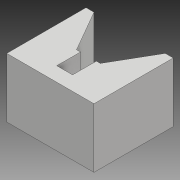
# Autodesk Inventor part: soporte_antena_aquiles
Saved by Autodesk Inventor 2018 (Build 220112000, 112)
## iProperties
Created: 2019-01-15
Part Number: soporte_antena_aquiles
Material: Genérico
Document SubType Name: Modeling
Designer: becar
Density: 1 g/cm^3
Appearance: Valor por defecto
Author: becar
Autodesk Inventor part; units mm, degrees
ref_plane "YZ Plane" through (0, 0, 0) normal (1, 0, 0) x (0, 1, 0)
ref_plane "XZ Plane" through (0, 0, 0) normal (0, 1, 0) x (-1, 0, 0)
ref_plane "XY Plane" through (0, 0, 0) normal (0, 0, 1) x (1, 0, 0)
sketch "Boceto1" plane through (0, 0, 0) normal (0, 0, 1) x (1, 0, 0)
  line L0 (0, 0) -> (0, 15)
  line L1 (0, 15) -> (2, 15)
  line L2 (2, 15) -> (8, 4.6077)
  line L3 (2, 15) -> (14, 15) construction
  line L4 (0, 0) -> (0, -5)
  line L5 (8, 4.6077) -> (14, 4.6077)
  line L6 (14, 4.6077) -> (20, 15)
  line L7 (20, 15) -> (22, 15)
  line L8 (22, 15) -> (22, -0.0111)
  line L9 (22, -0.0111) -> (22, -5)
  line L10 (22, -5) -> (0, -5)
  dimension "d0" = 15
  dimension "d1" = 2
  dimension "d2" = 12
  dimension "d3" = 60
  dimension "d4" = 5
  dimension "d5" = 6
  dimension "d6" = 12
  dimension "d7" = 2
  constraints: 22 end point, 3 perpendicular, 2 horizontal, 2 vertical, 1 equal length, 1 parallel, 1 point on line
  measures "d0" distance of L0.start L0.end
  measures "d1" distance of L0.end L1.end
  measures "d2" distance of L1.end L2.end
  measures "d3" angle of L2 L3
  measures "d4" distance of L0.start L4.end
  measures "d5" distance of L2.end L5.end
  measures "d6" distance of L5.end L6.end
  measures "d7" distance of L6.end L7.end
extrude "Extrusión1" add sketch "Boceto1" along normal blind 15
sketch "Boceto2" plane through (0, 0, 15) normal (0, 0, 1) x (1, 0, 0)
  line L0 (14, 4.6077) -> (8, 4.6077) projected
  line L1 (8, 4.6077) -> (9, 4.6077)
  line L2 (9, 4.6077) -> (9, -1.3923)
  line L3 (9, -1.3923) -> (13, -1.3923)
  line L4 (13, -1.3923) -> (13, 4.6077)
  line L5 (9, 4.6077) -> (13, 4.6077)
  point P0 (0, 0)
  dimension "d10" = 1
  dimension "d11" = 6
  dimension "d12" = 4
  constraints: 10 end point, 3 perpendicular, 2 point on line, 1 collinear
  measures "d10" distance of L0.end L1.end
  measures "d11" distance of L1.end L2.end
  measures "d12" distance of L2.end L3.end
extrude "Extrusión2" cut sketch "Boceto2" against normal blind 12
sketch "Boceto3" plane through (0, 0, 0) normal (0, 0, -1) x (-1, 0, 0)
  line L0 (-22, -5) -> (-22, 15) projected
  line L1 (-22, -5) -> (-22, 15)
  line L2 (-2, 15) -> (0, 15) projected
  line L3 (-22, 15) -> (0, 15)
  line L4 (0, 15) -> (0, -5) projected
  line L5 (0, 15) -> (0, -5)
  line L6 (0, -5) -> (-22, -5)
  line L7 (0, -5) -> (-22, -5) projected
  line L8 (-16.5, 0) -> (-15, 0)
  line L9 (-16.5, 0) -> (-18, 0)
  line L10 (-11, 11) -> (-12.5, 11)
  line L11 (-12.5, 11) -> (-18, 0)
  line L12 (-11, 11) -> (-9.5, 11)
  line L13 (-5.5, 0) -> (-7, 0)
  line L14 (-5.5, 0) -> (-4, 0)
  line L15 (-4, 0) -> (-9.5, 11)
  line L16 (-15, 0) -> (-14, 2)
  line L17 (-7, 0) -> (-8, 2)
  line L18 (-14, 2) -> (-8, 2)
  line L19 (-11, 4) -> (-10, 4)
  line L20 (-10, 4) -> (-9, 4)
  line L21 (-9, 4) -> (-11, 8)
  line L22 (-11, 4) -> (-13, 4)
  line L23 (-13, 4) -> (-11, 8)
  line L24 (-13, 4) -> (-11, 8)
  line L25 (-11, 8) -> (-9, 4)
  line L26 (-9, 4) -> (-13, 4)
  point P0 (0, 0)
  dimension "d16" = 1.5
  dimension "d23" = 1.5
  dimension "d24" = 1.5
  dimension "d25" = 1.5
  dimension "d26" = 3
  dimension "d27" = 4
  dimension "d29" = 1
  constraints: 46 end point, 5 collinear, 3 horizontal, 2 parallel, 2 point on line, 1 perpendicular
  measures "d16" distance of L8.start L9.end
  measures "d23" distance of L10.start L12.end
  measures "d24" distance of L13.start L13.end
  measures "d25" distance of L13.start L14.end
  measures "d26" distance of L10.start L21.end
  measures "d27" distance of L21.end L19.start
  measures "d29" distance of L19.start L19.end
extrude "Extrusión3" add sketch "Boceto3" against normal blind 3 contours L0 L3 L2 L4 L6 | L9 L11 L10 L12 L15 L14 L13 L17 L18 L16 L8 | L22 L23 L21 L20 L19
extrude "Extrusión4" cut sketch "Boceto3" against normal blind 1 contours L9 L11 L10 L12 L15 L14 L13 L17 L18 L16 L8
